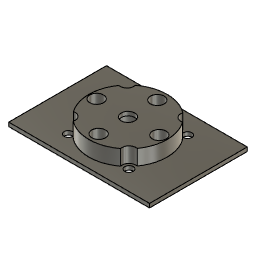
support_cam (Autodesk Fusion 360 design; units mm, degrees)
Autodesk Fusion 360 part; units mm, degrees
note: some values were not read from the file. Set by a fixed rule: which sketch regions a step uses.
sketch "Esquisse1" plane through (0, 0, 0) normal (0, 0, 1) x (1, 0, 0)
  line L0 (0, 25) -> (36, 25)
  line L1 (36, 25) -> (36, 0)
  line L2 (36, 0) -> (0, 0)
  line L3 (0, 0) -> (0, 25)
  line L4 (18, -4.4176) -> (18, 55.8936)
  circle A0 centre (10.25, 20) radius 1.075
  circle A1 centre (18, 20) radius 1.075
  line L5 (-6.2165, 12.5) -> (42, 12.5)
  circle A2 centre (9.9834, 12.5) radius 1.075
  circle A3 centre (25.75, 20) radius 1.075
  circle A4 centre (18, 20) radius 1.075
  circle A5 centre (26.0166, 12.5) radius 1.075
  circle A6 centre (10.25, 5) radius 1.075
  circle A7 centre (18, 5) radius 1.075
  circle A8 centre (25.75, 5) radius 1.075
  circle A9 centre (18, 12.5) radius 10
  circle A10 centre (18, 12.5) radius 1.75
  circle A11 centre (25.75, 20) radius 1.75
  circle A12 centre (18, 20) radius 1.75
  circle A13 centre (26.0166, 12.5) radius 1.75
  circle A14 centre (25.75, 5) radius 1.75
  circle A15 centre (18, 5) radius 1.75
  circle A16 centre (26.0166, 12.5) radius 1.75
  circle A17 centre (10.25, 20) radius 1.75
  circle A18 centre (9.9834, 12.5) radius 1.75
  circle A19 centre (10.25, 5) radius 1.75
  circle A20 centre (18, 12.5) radius 3
  point P0 (18, 12.5)
  dimension "d1" = 36
  dimension "d2" = 25
  dimension "d3" = 12.5
  dimension "d4" = 18
  dimension "d5" = 2.15
  dimension "d6" = 2.15
  dimension "d7" = 7.75
  dimension "d10" = 2.15
  dimension "d11" = 7.5
  dimension "d12" = 5
  dimension "d13" = 5
  dimension "d16" = 20
  dimension "d21" = 3.5
  dimension "d26" = 3.5
  dimension "d27" = 3.5
  dimension "d28" = 3.5
  dimension "d32" = 6
  constraint horizontal L0
  constraint vertical L1
  constraint horizontal L2
  constraint vertical L3
  constraint perpendicular L0 L4
  constraint coincident L4 A1.centre
  constraint perpendicular L4 L5
  constraint coincident L5 A2.centre
  constraint symmetric L4 A0 A3
  constraint symmetric L4 A1 A4
  constraint symmetric L4 A2 A5
  constraint symmetric A0 L5 A6
  constraint symmetric L5 A3 A8
  constraint symmetric L5 A4 A7
  constraint coincident P0 A9.centre
  constraint concentric A3 A11
  constraint concentric A1 A12
  constraint concentric A5 A13
  constraint symmetric L5 A11 A14
  constraint symmetric L5 A12 A15
  constraint symmetric L5 A13 A16
  constraint symmetric L4 A11 A17
  constraint symmetric L4 A14 A19
  constraint symmetric L4 A16 A18
  constraint concentric A9 A20
  measures "d1" distance of L0.start L0.end
  measures "d2" distance of L0.end L1.end
  measures "d3" distance of L0 P0
  measures "d4" distance of L3 P0
  measures "d5" diameter of A0
  measures "d6" diameter of A1
  measures "d7" horizontal distance of A0.centre A1.centre
  measures "d10" diameter of A2
  measures "d11" vertical distance of A0.centre A2.centre
  measures "d12" distance of L0 A0.centre
  measures "d13" distance of L0 A1.centre
  measures "d16" diameter of A9
  measures "d21" diameter of A10
  measures "d26" diameter of A11
  measures "d27" diameter of A12
  measures "d28" diameter of A13
  measures "d32" diameter of A20
extrude "Extrusion4" add sketch "Esquisse1" along normal blind 1 contours L0 L3 L4 L5 A9 A17 | L0 L1 L4 L5 A9 A11 | L2 L3 L4 L5 A9 A19 | L1 L2 L4 L5 A9 A14 | A3 A9 A11 | A0 A9 A17 | A6 A9 A19 | A8 A9 A14 picked at (24.3887, 20.4618) picked at (11.6014, 20.4841) picked at (11.6014, 4.5159) picked at (24.3887, 4.5382)
extrude "Extrusion5" add sketch "Esquisse1" along normal blind 4.9 contours L4 L5 A9 A11 A12 A13 A16 A20 | L4 L5 A9 A12 A17 A18 A20 | L4 L5 A9 A15 A18 A19 A20 | L4 A1 A4 A12 | L4 A1 A4 A12 | A3 A9 A11 | A0 A9 A17 | L5 A2 A18 | L5 A2 A18 | A6 A9 A19 | L4 L5 A9 A13 A14 A15 A16 A20 | L5 A5 A13 A16 | L5 A5 A13 A16 | A8 A9 A14 | L4 L5 A10 A20 | L4 L5 A10 A20 | L4 A7 A15 | L4 A7 A15 | L4 L5 A10 A20 | L4 L5 A10 A20 picked at (25.5724, 18.6548) picked at (10.4124, 18.6517) picked at (10.4124, 6.3483) picked at (24.3997, 5.1334)
extrude "Extrusion6" cut sketch "Esquisse1" along normal blind 5 from surface at 1 contours L4 A1 A4 A12 | L4 A1 A4 A12 | A3 A9 A11 | A3 A9 A11 | A0 A9 A17 | A0 A9 A17 | L5 A2 A18 | L5 A2 A18 | A6 A9 A19 | A6 A9 A19 | L5 A5 A13 A16 | L5 A5 A13 A16 | A8 A9 A14 | A8 A9 A14 | L4 A7 A15 | L4 A7 A15
extrude "Extrusion8" cut sketch "Esquisse1" along normal blind 3.9 contours L4 L5 A10 A20 | L4 L5 A10 A20 | L4 L5 A10 A20 | L4 L5 A10 A20
extrude "Extrusion7" [suppressed]
